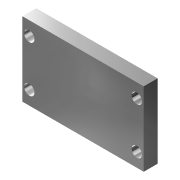
# Autodesk Inventor part: suporte-barra
Saved by Autodesk Inventor 2015 (Build 190159000, 159)
## iProperties
Created: 2016-08-11
Part Number: suporte-barra
Material: Steel, Carbon
Document SubType Name: Modeling
Designer: EriveltonDell
Density: 7.87 g/cm^3
Appearance: Chrome - Polished
Mass: 377.778 g
Surface Area: 137.801 cm^2
Volume: 48.0022 cm^3
Author: EriveltonDell
Autodesk Inventor part; units mm, degrees
ref_plane "YZ Plane" through (0, 0, 0) normal (1, 0, 0) x (0, 1, 0)
ref_plane "XZ Plane" through (0, 0, 0) normal (0, 1, 0) x (-1, 0, 0)
ref_plane "XY Plane" through (0, 0, 0) normal (0, 0, 1) x (1, 0, 0)
sketch "Sketch11" plane through (0, 0, 0) normal (0, 1, 0) x (-1, 0, 0)
  line L0 (0, 0) -> (52.5, 0)
  line L1 (52.5, 0) -> (52.5, 32)
  line L2 (52.5, 32) -> (0, 32)
  line L3 (0, 32) -> (0, 0)
  line L4 (52.5, 32) -> (49.5, 32)
  dimension "d63" = 52.5
  dimension "d64" = 32
  dimension "d67" = 3
  constraints: 10 end point, 2 parallel, 1 horizontal, 1 perpendicular, 1 point on line
  measures "d63" distance of L2.end L1.end
  measures "d64" distance of L1.end L0.end
  measures "d67" distance of L1.end L4.end
extrude "Extrusion10" add sketch "Sketch11" along normal blind 6
sketch "Sketch12" plane through (0, 0, 0) normal (0, -1, 0) x (1, 0, 0)
  line L0 (-52.5, 32) -> (-49.5, 32)
  line L1 (-52.5, 32) -> (0, 32) projected
  line L2 (-49.5, 32) -> (-49.5, 26)
  circle A0 centre (-49.5, 26) radius 2.25
  circle A1 centre (-3, 26) radius 2.25
  circle A2 centre (-49.5, 6) radius 2.25
  circle A3 centre (-3, 6) radius 2.25
  point P0 (0, 0)
  dimension "d68" = 3
  dimension "d69" = 6
  dimension "d70" = 4.5
  dimension "d73" = 46.5
  dimension "d76" = 20
  constraints: 4 centre point, 4 end point, 1 coincident, 1 horizontal, 1 perpendicular, 1 point on line, 1 vertical, 6 other
  measures "d68" distance of L0.start L0.end
  measures "d69" distance of L0.end L2.end
  measures "d70" diameter of A0
  measures "d73" distance of A0.centre A1.centre
  measures "d76" distance of A0.centre A2.centre
extrude "Extrusion11" cut sketch "Sketch12" against normal blind 10
body "Solid2"
